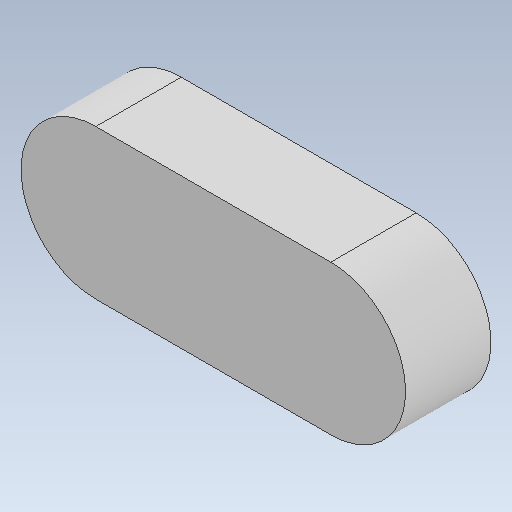
# Autodesk Inventor part: key2
Saved by Autodesk Inventor 2020 (Build 240168000, 168)
## iProperties
Created: 2021-06-15
Part Number: key2
Material: 常规
Document SubType Name: Modeling
Designer: dell
Density: 1 g/cm^3
Appearance: 默认
Author: dell
Autodesk Inventor part; units mm, degrees
ref_plane "YZ Plane" through (0, 0, 0) normal (1, 0, 0) x (0, 1, 0)
ref_plane "XZ Plane" through (0, 0, 0) normal (0, 1, 0) x (-1, 0, 0)
ref_plane "XY Plane" through (0, 0, 0) normal (0, 0, 1) x (1, 0, 0)
sketch "草图1" plane through (0, 0, 0) normal (0, 0, 1) x (1, 0, 0)
  line L0 (-11, 1) -> (11, 1) projected
  arc A0 (-11, 1) -> (-11, -13) centre (-11, -6) ccw projected
  line L1 (-11, -13) -> (11, -13) projected
  arc A1 (11, -13) -> (11, 1) centre (11, -6) ccw projected
  line L2 (-11, -6) -> (11, -6) construction
  line L3 (-11, -13) -> (11, -13)
  line L4 (11, 1) -> (-11, 1)
  arc A2 (-11, 1) -> (-11, -13) centre (-11, -6) ccw
  arc A3 (11, -13) -> (11, 1) centre (11, -6) ccw
  point P0 (0, 0)
  point P1 (0, -6)
  constraints: 8 end point, 4 point on circle, 4 tangent, 2 centre point, 1 concentric, 1 horizontal, 1 midpoint, 1 parallel, 1 other
extrude "拉伸1" add sketch "草图1" along normal blind 8
